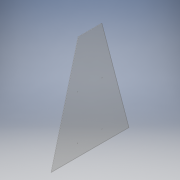
# Autodesk Inventor part: Polycarb Side Pannel
Saved by Autodesk Inventor 2016 (Build 200138000, 138)
## iProperties
Created: 2018-05-16
Part Number: Polycarb Side Pannel
Material: Polycarbonate, Clear
Document SubType Name: Modeling
Designer: Kade
Density: 1.2 g/cm^3
Appearance: Polycarbonate - Clear
Mass: 1475.73 g
Surface Area: 7834.71 cm^2
Volume: 1229.78 cm^3
Author: Kade
Autodesk Inventor part; units mm, degrees
ref_plane "YZ Plane" through (0, 0, 0) normal (1, 0, 0) x (0, 1, 0)
ref_plane "XZ Plane" through (0, 0, 0) normal (0, 1, 0) x (-1, 0, 0)
ref_plane "XY Plane" through (0, 0, 0) normal (0, 0, 1) x (1, 0, 0)
sketch "Sketch1" plane through (0, 0, 0) normal (1, 0, 0) x (0, 1, 0)
  line L0 (0, 0) -> (0, 666.8516)
  line L1 (0, 333.4258) -> (890.5513, 333.4258) construction
  line L2 (890.5513, 435.0258) -> (890.5513, 333.4258)
  line L3 (890.5513, 333.4258) -> (890.5513, 231.8258)
  line L4 (890.5513, 435.0258) -> (0, 666.8516)
  line L5 (890.5513, 231.8258) -> (0, 0)
  dimension "d0" = 666.8516
  dimension "d4" = 203.2
  dimension "d6" = 920.2309
  dimension "d7" = 920.2309
  dimension "d10" = 180
  constraints: 12 end point, 2 vertical, 1 horizontal, 1 midpoint
  measures "d0" distance of L0.start L0.end
  measures "d4" distance of L3.end L2.start
  measures "d6" distance of L2.start L0.end
  measures "d7" distance of L3.end L0.start
  measures "d10" angle of L3 L2
extrude "Extrusion1" add sketch "Sketch1" along normal blind 3.175
sketch "Sketch2" plane through (3.175, 0, 0) normal (1, 0, 0) x (0, 0, -1)
  circle A0 centre (-231.8258, 482.6) radius 2.5527
  circle A1 centre (-435.0258, 482.6) radius 2.5527
  circle A2 centre (-231.8258, 101.6) radius 2.5527
  circle A3 centre (-435.0258, 101.6) radius 2.5527
  line L0 (-666.8516, 0) -> (0, 0) projected
  dimension "d11" = 5.1054
  dimension "d12" = 5.1054
  dimension "d13" = 203.2
  dimension "d14" = 5.1054
  dimension "d15" = 5.1054
  dimension "d16" = 203.2
  dimension "d17" = 0
  dimension "d18" = 381
  dimension "d19" = 101.6
  dimension "d20" = 231.8258
  dimension "d21" = 231.8258
  dimension "d24" = 0
  constraints: 4 centre point
  measures "d11" diameter of A0
  measures "d12" diameter of A1
  measures "d13" distance of A0.centre A1.centre
  measures "d14" diameter of A2
  measures "d15" diameter of A3
  measures "d16" distance of A2.centre A3.centre
  measures "d17" vertical distance of A3.centre A2.centre
  measures "d18" distance of A1.centre A3.centre
  measures "d19" distance from line of L0 A2.centre
  measures "d20" horizontal distance of L0.end A2.centre
  measures "d21" horizontal distance of L0.start A3.centre
  measures "d24" horizontal distance of A2.centre A0.centre
extrude "Extrusion2" cut sketch "Sketch2" against normal blind 25.4
equation "\"d20\" = d21"
body "Solid1"
